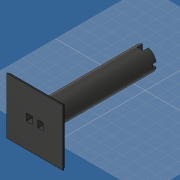
# Autodesk Inventor part: DayLightGlow_Rod
Saved by Autodesk Inventor 2019 (Build 230136000, 136)
## iProperties
Created: 2019-01-01
Part Number: DayLightGlow_Rod
Material: Generisch
Document SubType Name: Modeling
Designer: Stefan
Mass: 227.283 g
Surface Area: 626.544 cm^2
Volume: 227.283 cm^3
Density: 1 g/cm^3
Appearance: Glatt - Schwarz
Author: Stefan
Autodesk Inventor part; units mm, degrees
ref_plane "YZ Plane" through (0, 0, 0) normal (1, 0, 0) x (0, 1, 0)
ref_plane "XZ Plane" through (0, 0, 0) normal (0, 1, 0) x (-1, 0, 0)
ref_plane "XY Plane" through (0, 0, 0) normal (0, 0, 1) x (1, 0, 0)
sketch "Skizze1" plane through (0, 0, 0) normal (0, 0, 1) x (1, 0, 0)
  line L0 (-14, 6.25) -> (-5, 6.25)
  line L1 (-4, 5.25) -> (-4, -5.25)
  line L2 (-5, -6.25) -> (-14, -6.25)
  line L3 (-15, -5.25) -> (-15, 5.25)
  line L4 (-15, 6.25) -> (-4, -6.25) construction
  line L5 (-4, 6.25) -> (-15, -6.25) construction
  line L6 (6.5, 6.25) -> (14, 6.25)
  line L7 (15, 5.25) -> (15, -5.25)
  line L8 (14, -6.25) -> (6.5, -6.25)
  line L9 (5.5, -5.25) -> (5.5, 5.25)
  line L10 (5.5, 6.25) -> (15, -6.25) construction
  line L11 (15, 6.25) -> (5.5, -6.25) construction
  arc A0 (-15, -5.25) -> (-14, -6.25) centre (-14, -5.25) ccw
  arc A1 (-14, 6.25) -> (-15, 5.25) centre (-14, 5.25) ccw
  arc A2 (-4, 5.25) -> (-5, 6.25) centre (-5, 5.25) ccw
  arc A3 (-5, -6.25) -> (-4, -5.25) centre (-5, -5.25) ccw
  arc A4 (6.5, 6.25) -> (5.5, 5.25) centre (6.5, 5.25) ccw
  arc A5 (15, 5.25) -> (14, 6.25) centre (14, 5.25) ccw
  arc A6 (14, -6.25) -> (15, -5.25) centre (14, -5.25) ccw
  arc A7 (5.5, -5.25) -> (6.5, -6.25) centre (6.5, -5.25) ccw
  line L12 (-4, 4.5) -> (5.5, 4.5)
  line L13 (5.5, 4.5) -> (5.5, -4.5)
  line L14 (5.5, -4.5) -> (-4, -4.5)
  line L15 (-4, -4.5) -> (-4, 4.5)
  circle A8 centre (0, 0) radius 20
  line L16 (-15.25, -6.75) -> (15.25, -6.75)
  line L17 (15.25, -6.75) -> (15.25, 6.75)
  line L18 (15.25, 6.75) -> (-15.25, 6.75)
  line L19 (-15.25, 6.75) -> (-15.25, -6.75)
  line L20 (-15.25, -6.75) -> (15.25, 6.75) construction
  line L21 (15.25, -6.75) -> (-15.25, 6.75) construction
  line L22 (0, 6.75) -> (0, -6.75) construction
  line L23 (-28, 0) -> (28, 0) projected
  circle A9 centre (0, 0) radius 15 construction
  line L24 (10.6066, 10.6066) -> (-10.6066, -10.6066) construction
  line L25 (-10.6066, 10.6066) -> (10.6066, -10.6066) construction
  line L26 (6, 20) -> (-4.5, 20)
  line L27 (-4.5, 20) -> (-4.5, 4.5)
  line L28 (-4.5, 4.5) -> (6, 4.5)
  line L29 (6, 4.5) -> (6, 20)
  line L30 (20, 4) -> (15.25, 4)
  line L31 (15.25, 4) -> (15.25, -4)
  line L32 (15.25, -4) -> (20, -4)
  line L33 (20, -4) -> (20, 4)
  line L34 (-15.25, 4) -> (-20, 4)
  line L35 (-20, 4) -> (-20, -4)
  line L36 (-20, -4) -> (-15.25, -4)
  line L37 (-15.25, -4) -> (-15.25, 4)
  point P0 (-9.5, 0)
  point P1 (10.25, 0)
  point P2 (-9.5, 0)
  point P3 (10.25, 0)
  point P4 (-9.5, 0)
  point P5 (-4, 0)
  point P6 (5.5, 0)
  point P7 (10.25, 0)
  point P8 (0.75, 4.5)
  point P9 (0, 0)
  point P10 (0.75, 20)
  dimension "d5" = 12.5
  dimension "d6" = 11
  dimension "d7" = 9.5
  dimension "d9" = 1
  dimension "d10" = 1
  dimension "d12" = 9
  dimension "d14" = 40
  dimension "d15" = 13.5
  dimension "d16" = 30.5
  dimension "d17" = 30
  dimension "d18" = 9.5
  dimension "d47" = 30
  dimension "d48" = 90
  dimension "d49" = 45
  dimension "d50" = 10.5
  dimension "d55" = 8
  constraints: 74 end point, 20 midpoint, 20 point on circle, 20 point on line, 19 tangent, 16 parallel, 10 centre point, 7 horizontal, 7 perpendicular, 6 equal radius, 4 collinear, 3 coincident, 3 horizontal alignment, 1 vertical alignment, 2 other
  measures "d5" distance between parallel lines of L2 L0
  measures "d6" distance between parallel lines of L1 L3
  measures "d7" distance between parallel lines of L7 L9
  measures "d9" radius of A0
  measures "d10" radius of A4
  measures "d12" distance between parallel lines of L14 L12
  measures "d14" diameter of A8
  measures "d15" distance between parallel lines of L16 L18
  measures "d16" distance between parallel lines of L17 L19
  measures "d17" distance between parallel lines of L7 L3
  measures "d18" distance between parallel lines of L9 L15
  measures "d47" diameter of A9
  measures "d48" angle of L24 L25
  measures "d49" angle of L22 L24
  measures "d50" distance of L26.start L26.end
  measures "d55" distance between parallel lines of L32 L30
extrude "Extrusion1" add sketch "Skizze1" along normal blind 194.899 contours A1 L3 L23 L19 L18 L27 A2 L0 | L27 L18 L29 A4 L9 L12 L1 A2 | L3 A0 L2 A3 L1 L14 L9 A7 L8 A6 L7 L23 L17 L16 L19 | L27 A8 L29 L18 | L18 L19 L34 A8 L27 | L23 A8 L34 L19 | L19 L36 A8 L23 | L23 L9 L14 L1 | L1 L12 L9 L23 | L29 A8 L30 L17 L18 | L18 L17 L23 L7 A5 L6 A4 L29 | L19 L16 L17 L32 A8 L36 | L30 A8 L23 L17 | L32 L17 L23 A8
extrude "Extrusion4" cut sketch "Skizze1" along normal blind 10 contours A1 L3 L23 L19 L18 L27 A2 L0 | L27 L18 L29 A4 L9 L12 L1 A2 | A2 L1 L28 L27 | L3 A0 L2 A3 L1 L14 L9 A7 L8 A6 L7 L23 L17 L16 L19 | L27 A8 L29 L18 | L23 L9 L14 L1 | L1 L12 L9 L23 | L18 L17 L23 L7 A5 L6 A4 L29 | L27 L26 A8 | L9 A4 L29 L28 | A8 L26 L29
extrude "Extrusion6" cut sketch "Skizze1" along normal blind 17 contours L23 L9 L14 L1 | L1 L12 L9 L23
extrude "Extrusion5" cut sketch "Skizze1" along normal blind 6 contours L23 A8 L34 L19 | L19 L36 A8 L23 | L35 L34 A8 | A8 L36 L35 | L30 A8 L23 L17 | L30 L33 A8 | L32 L17 L23 A8 | A8 L33 L32
sketch "Skizze2" plane through (0, 0, 194.899) normal (0, 0, 1) x (1, 0, 0)
  arc A0 (-15, -5.25) -> (-14, -6.25) centre (-14, -5.25) ccw projected
  line L0 (-15, -5.25) -> (-15, 5.25) projected
  arc A1 (-14, 6.25) -> (-15, 5.25) centre (-14, 5.25) ccw projected
  line L1 (-14, 6.25) -> (-5, 6.25) projected
  arc A2 (-4, 5.25) -> (-5, 6.25) centre (-5, 5.25) ccw projected
  line L2 (-4, 5.25) -> (-4, -5.25) projected
  arc A3 (-5, -6.25) -> (-4, -5.25) centre (-5, -5.25) ccw projected
  line L3 (-5, -6.25) -> (-14, -6.25) projected
  arc A4 (6.5, 6.25) -> (5.5, 5.25) centre (6.5, 5.25) ccw projected
  line L4 (6.5, 6.25) -> (14, 6.25) projected
  arc A5 (15, 5.25) -> (14, 6.25) centre (14, 5.25) ccw projected
  line L5 (15, 5.25) -> (15, -5.25) projected
  arc A6 (14, -6.25) -> (15, -5.25) centre (14, -5.25) ccw projected
  line L6 (14, -6.25) -> (6.5, -6.25) projected
  arc A7 (5.5, -5.25) -> (6.5, -6.25) centre (6.5, -5.25) ccw projected
  line L7 (5.5, -5.25) -> (5.5, 5.25) projected
  circle A8 centre (0, 0) radius 20 projected
  line L8 (-50, -50) -> (50, -50)
  line L9 (50, -50) -> (50, 50)
  line L10 (50, 50) -> (-50, 50)
  line L11 (-50, 50) -> (-50, -50)
  line L12 (-50, -50) -> (50, 50) construction
  line L13 (50, -50) -> (-50, 50) construction
  line L14 (-48.8, 48.8) -> (48.8, 48.8)
  line L15 (48.8, 48.8) -> (48.8, -48.8)
  line L16 (48.8, -48.8) -> (-48.8, -48.8)
  line L17 (-48.8, -48.8) -> (-48.8, 48.8)
  dimension "d19" = 100
  dimension "d20" = 100
  dimension "d21" = 1.2
  constraints: 20 end point, 4 parallel, 2 midpoint, 2 perpendicular, 1 horizontal, 3 other
  measures "d19" distance of L9.end L10.end
  measures "d20" distance of L10.end L8.start
  measures "d21" distance between parallel lines of L14 L10
extrude "Extrusion2" add sketch "Skizze2" along normal blind 2 contours A8 | L11 L10 L9 L8 | L14 L15 L16 L17
extrude "Extrusion3" add sketch "Skizze2" against normal blind 2 contours L14 L15 L16 L17
hole "Bohrung1" at (10.6066, 10.6066, 0) at (-10.6066, 10.6066, 0) at (-10.6066, -10.6066, 0) at (10.6066, -10.6066, 0) direction (0, 0, 1) diameter 2.2 depth 5
sketch "Skizze3" plane through (0, 0, 0) normal (0, 1, 0) x (-1, 0, 0)
  line L0 (20, 12) -> (20.5, 12)
  line L1 (20.5, 12) -> (20.5, 0)
  line L2 (20.5, 0) -> (20, 0)
  line L3 (20, 0) -> (20, 12)
  line L4 (20.6, 0) -> (19.9, 0) projected
  line L5 (0, -2.4) -> (0, 14.4) projected
  dimension "d26" = 12
  dimension "d27" = 0.5
  dimension "d37" = 40
  constraints: 8 end point, 2 parallel, 1 collinear, 1 horizontal, 1 perpendicular
  measures "d26" distance of L2.end L0.start
  measures "d27" distance between parallel lines of L1 L3
  measures "d37" diameter of L3 L5
equation "\"d20\" = d19"
